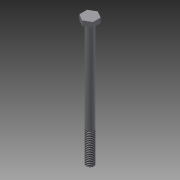
# Autodesk Inventor part: mechanical stop bolt
Saved by Autodesk Inventor 2015 SP1 (Build 190203100, 203)
## iProperties
Created: 2015-01-28
Part Number: mechanical stop bolt
Material: Generic
Document SubType Name: Modeling
Designer: Admin
Density: 1 g/cm^3
Appearance: Default
Author: Admin
Autodesk Inventor part; units mm, degrees
ref_plane "YZ Plane" through (0, 0, 0) normal (1, 0, 0) x (0, 1, 0)
ref_plane "XZ Plane" through (0, 0, 0) normal (0, 1, 0) x (-1, 0, 0)
ref_plane "XY Plane" through (0, 0, 0) normal (0, 0, 1) x (1, 0, 0)
sketch "Sketch1" plane through (0, 0, 0) normal (0, 1, 0) x (-1, 0, 0)
  circle A0 centre (0, 0) radius 3.175
  dimension "d0" = 6.35
  constraints: 1 centre point, 1 coincident
  measures "d0" diameter of A0
extrude "Extrusion1" add sketch "Sketch1" along normal blind 101.6
sketch "Sketch2" plane through (0, 101.6, 0) normal (0, 1, 0) x (1, 0, 0)
  circle A0 centre (0, 0) radius 3.175 projected
  line L0 (-5.5563, -3.2079) -> (-5.5563, 3.2079)
  line L1 (-5.5563, 3.2079) -> (0, 6.4158)
  line L2 (0, 6.4158) -> (5.5563, 3.2079)
  line L3 (5.5563, 3.2079) -> (5.5563, -3.2079)
  line L4 (5.5563, -3.2079) -> (0, -6.4158)
  line L5 (0, -6.4158) -> (-5.5563, -3.2079)
  dimension "d3" = 11.1125
  dimension "d4" = 11.1125
  dimension "d5" = 11.1125
  dimension "d6" = 120
  dimension "d7" = 120
  dimension "d8" = 5.5563
  dimension "d9" = 5.5563
  dimension "d10" = 5.5563
  constraints: 12 end point, 3 parallel, 1 vertical
  measures "d3" distance between parallel lines of L3 L0
  measures "d4" distance between parallel lines of L4 L1
  measures "d5" distance between parallel lines of L2 L5
  measures "d6" angle of L0 L5
  measures "d7" angle of L1 L0
  measures "d8" distance from line of A0.centre L0
  measures "d9" distance from line of L1 A0.centre
  measures "d10" distance from line of L5 A0.centre
extrude "Extrusion2" add sketch "Sketch2" along normal blind 3.9688 contours A0 | L0 L1 L2 L3 L4 L5
thread "Thread1" size "1/4-20 UNC" class "2A" standard "ANSI Unified Screw Threads" length 25.4 offset 76.2
body "Solid1"
